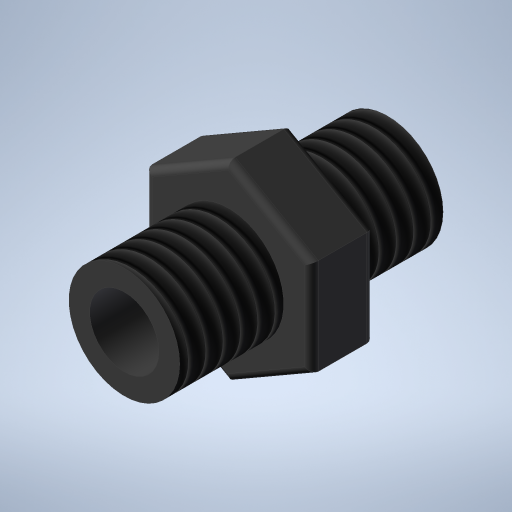
# Autodesk Inventor part: HUDSON-1-82
Saved by Autodesk Inventor 2024.2 (Build 282272000, 272)
## iProperties
Created: 2024-10-06
Part Number: HUDSON-1-82
Material: Generic
Document SubType Name: Modeling
Designer: melim
Density: 1 g/cm^3
Appearance: Default
Author: melim
Autodesk Inventor part; units mm, degrees
ref_plane "YZ Plane" through (0, 0, 0) normal (1, 0, 0) x (0, 1, 0)
ref_plane "XZ Plane" through (0, 0, 0) normal (0, 1, 0) x (-1, 0, 0)
ref_plane "XY Plane" through (0, 0, 0) normal (0, 0, 1) x (1, 0, 0)
sketch "Sketch1" plane through (0, 0, 0) normal (0, 0, 1) x (1, 0, 0)
  line L0 (0, -6.9282) -> (-6, -3.4641)
  line L1 (-6, -3.4641) -> (-6, 3.4641)
  line L2 (-6, 3.4641) -> (0, 6.9282)
  line L3 (0, 6.9282) -> (6, 3.4641)
  line L4 (6, 3.4641) -> (6, -3.4641)
  line L5 (6, -3.4641) -> (0, -6.9282)
  circle A0 centre (0, 0) radius 4
  dimension "d0" = 12
  dimension "d1" = 8
  constraints: 12 end point, 2 coincident, 1 centre point, 13 other
  measures "d0" distance between parallel lines of L5 L2
  measures "d1" diameter of A0
extrude "Extrusion1" add sketch "Sketch1" along normal mid plane 4.5 contours L0 L1 L2 L3 L4 L5 | A0
extrude "Extrusion2" add sketch "Sketch1" along normal mid plane 18.5 contours A0
thread "Thread1" size "M8x1.25" class "6g" standard "ANSI Metric M Profile" full length
sketch "Sketch2" plane through (0, 0, -9.25) normal (0, 0, -1) x (-1, 0, 0)
  point P0 (0, 0)
hole "Hole1" at (0, 0, -9.25) direction (0, 0, 1) diameter 5 end through all
fillet "Fillet1" radius 0.5 12 edges at (-6, 0, -2.25) (-3, -5.1962, -2.25) (3, -5.1962, -2.25) (-3, 5.1962, -2.25) (6, 0, -2.25) (3, 5.1962, -2.25) (-3, 5.1962, 2.25) (3, 5.1962, 2.25) (6, 0, 2.25) (3, -5.1962, 2.25) (-3, -5.1962, 2.25) (-6, 0, 2.25)
sketch "Sketch3" plane through (0, 0, 9.25) normal (0, 0, 1) x (1, 0, 0)
  circle A0 centre (0, 0) radius 4
  circle A1 centre (0, 0) radius 2.5
  dimension "d16" = 8
  dimension "d17" = 5
  constraints: 2 centre point, 2 coincident
  measures "d16" diameter of A0
  measures "d17" diameter of A1
extrude "Extrusion3" add sketch "Sketch3" along normal blind 0.5
thread "Thread2" size "M8x1.25" class "6g" standard "ANSI Metric M Profile" full length
body "Solid1"
